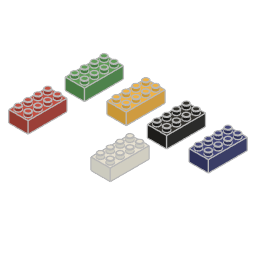
Toy blocks (Autodesk Fusion 360 design; units mm, degrees)
Autodesk Fusion 360 part; units mm, degrees
sketch "Sketch1" plane through (0, 0, 0) normal (0, 1, 0) x (1, 0, 0) in component "2x8 block"
  line L0 (0, 0) -> (-15.8, 0)
  line L1 (-15.8, 0) -> (-15.8, 31.8)
  line L2 (-15.8, 31.8) -> (0, 31.8)
  line L3 (0, 31.8) -> (0, 0)
  dimension "d1" = 15.8
  dimension "d2" = 31.8
  constraint horizontal L0
  constraint vertical L1
  constraint horizontal L2
  constraint vertical L3
  constraint coincident L0.start L3.end
  measures "d1" distance of L0.start L0.end
  measures "d2" distance of L0.start L2.end
extrude "Extrude1" add sketch "Sketch1" along normal blind 9.6 makes body 1 in component "2x8 block"
sketch "Sketch2" plane through (0, 9.6, 0) normal (0, 1, 0) x (-1, 0, 0) in component "2x8 block"
  line L0 (0, -31.8) -> (15.8, -31.8)
  line L1 (15.8, -31.8) -> (15.8, 0)
  line L2 (15.8, 0) -> (0, 0)
  line L3 (0, 0) -> (0, -31.8)
  circle A0 centre (11.9, -3.9) radius 2.5
  dimension "d5" = 5
  dimension "d6" = 3.9
  dimension "d7" = 3.9
  measures "d5" diameter of A0
  measures "d6" distance of L1 A0.centre
  measures "d7" distance of L2 A0.centre
extrude "Extrude2" add sketch "Sketch2" along normal blind 3 contours A0 bodies 1 in component "2x8 block"
pattern_linear "R-Pattern1" count 2 spacing 8 along (1, 0, 0) count 4 spacing 8 along (0, 0, -1) of "Extrude2" in component "2x8 block"
shell "Shell1" thickness 1.49 removed faces 1 at (-5.2667, 0, -21.2) on bodies 1 in component "2x8 block"
sketch "Sketch3" plane through (0, 8.11, 0) normal (0, -1, 0) x (1, 0, 0) in component "2x8 block"
  circle A0 centre (-3.9, -27.9) radius 1.01
  circle A1 centre (-11.9, -27.9) radius 1.01
  circle A2 centre (-3.9, -19.9) radius 1.01
  circle A3 centre (-11.9, -19.9) radius 1.01
  circle A4 centre (-3.9, -11.9) radius 1.01
  circle A5 centre (-11.9, -11.9) radius 1.01
  circle A6 centre (-3.9, -3.9) radius 1.01
  circle A7 centre (-11.9, -3.9) radius 1.01
  line L0 (-14.31, -30.31) -> (-1.49, -30.31)
  line L1 (-1.49, -30.31) -> (-1.49, -1.49)
  line L2 (-1.49, -1.49) -> (-14.31, -1.49)
  line L3 (-14.31, -1.49) -> (-14.31, -30.31)
  line L4 (-11.9, -11.9) -> (-3.9, -3.9) construction
  circle A8 centre (-7.9, -7.9) radius 3.15
  circle A9 centre (-7.9, -7.9) radius 2.15
  dimension "d15" = 6.3
  dimension "d16" = -1
  constraint coincident A5.centre L4.start
  constraint coincident A6.centre L4.end
  constraint midpoint L4 A8.centre
  measures "d15" diameter of A8
extrude "Extrude3" add sketch "Sketch3" along normal blind 8.1 contours A8 bodies 1 in component "2x8 block"
pattern_linear "R-Pattern2" count 3 spacing 8 along (0, 0, -1) of "Extrude3" in component "2x8 block"
fillet "Fillet1" radius 0.3 8 edges at (-9.5692, 12.6, -20.804) (-9.5692, 12.6, -12.804) (-9.5692, 12.6, -4.804) (-1.5692, 12.6, -4.804) (-1.5692, 12.6, -12.804) (-1.5692, 12.6, -20.804) (-1.5692, 12.6, -28.804) (-9.5692, 12.6, -28.804) on bodies 1 in component "2x8 block"
copy_body "CopyPasteBodies1" bodies 1 makes body 2
move_body "Move1" bodies 2 to x (1, 0, 0) y (0, 1, 0) z (0, 0, 1) at (0, 0, 46)
copy_body "CopyPasteBodies2" bodies 1 makes body 3
move_body "Move2" bodies 3 to x (1, 0, 0) y (0, 1, 0) z (0, 0, 1) at (34, 0, 0)
copy_body "CopyPasteBodies3" bodies 2 3 1 makes body 4 makes body 5 makes body 6
move_body "Move3" bodies 4 5 6 to x (1, 0, 0) y (0, 1, 0) z (0, 0, 1) at (67, 0, 0)
component "2x8 block" placed x (1, 0, 0) y (0, 1, 0) z (0, 0, 1) at (0, 0, 0)
